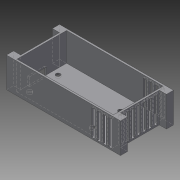
# Autodesk Inventor part: case body
Saved by Autodesk Inventor 2015 (Build 190159000, 159)
## iProperties
Created: 2019-05-19
Part Number: case body
Material: Generic
Document SubType Name: Modeling
Designer: Toby
Density: 1 g/cm^3
Appearance: Default
Author: Toby
Autodesk Inventor part; units mm, degrees
ref_plane "YZ Plane" through (0, 0, 0) normal (1, 0, 0) x (0, 1, 0)
ref_plane "XZ Plane" through (0, 0, 0) normal (0, 1, 0) x (-1, 0, 0)
ref_plane "XY Plane" through (0, 0, 0) normal (0, 0, 1) x (1, 0, 0)
sketch "Sketch1" plane through (0, 0, 0) normal (0, 0, 1) x (1, 0, 0)
  line L0 (-48.8389, 19.9623) -> (19.1611, 19.9623)
  line L1 (19.1611, 19.9623) -> (19.1611, -15.0377)
  line L2 (19.1611, -15.0377) -> (-48.8389, -15.0377)
  line L3 (-48.8389, -15.0377) -> (-48.8389, 19.9623)
  line L4 (-50.0389, 21.1623) -> (20.3611, 21.1623)
  line L5 (20.3611, 21.1623) -> (20.3611, -16.2377)
  line L6 (20.3611, -16.2377) -> (-50.0389, -16.2377)
  line L7 (-50.0389, -16.2377) -> (-50.0389, 21.1623)
  point P0 (0, 0)
  dimension "d0" = 35
  dimension "d1" = 68
  dimension "d2" = 1.2
  dimension "d3" = 1.2
  dimension "d4" = 1.2
  dimension "d5" = 1.2
  constraints: 16 end point, 4 parallel, 2 horizontal, 2 perpendicular
  measures "d0" distance between parallel lines of L2 L0
  measures "d1" distance of L0.start L0.end
  measures "d2" distance between parallel lines of L0 L4
  measures "d3" distance between parallel lines of L6 L2
  measures "d4" distance between parallel lines of L7 L3
  measures "d5" distance between parallel lines of L1 L5
extrude "Extrusion1" add sketch "Sketch1" along normal blind 20
sketch "Sketch2" plane through (0, 0, 0) normal (0, 0, -1) x (-1, 0, 0)
  line L0 (-20.3611, 21.1623) -> (50.0389, 21.1623)
  line L1 (50.0389, 21.1623) -> (50.0389, -16.2377)
  line L2 (50.0389, -16.2377) -> (-20.3611, -16.2377)
  line L3 (-20.3611, -16.2377) -> (-20.3611, 21.1623)
  point P0 (0, 0)
  constraints: 8 end point, 2 parallel, 1 horizontal, 1 perpendicular
extrude "Extrusion2" add sketch "Sketch2" along normal blind 1.2
sketch "Sketch3" plane through (-50.0389, -16.2377, 20) normal (-1, 0, 0) x (0, 0, 1)
  line L0 (-21.2, 0) -> (-21.2, 37.4) projected
  line L1 (-21.2, 22) -> (-15.2, 22)
  line L2 (-15.2, 22) -> (-15.2, 10)
  line L3 (-15.2, 10) -> (-21.2, 10)
  line L4 (-21.2, 10) -> (-21.2, 22)
  line L5 (0, 0) -> (-21.2, 0) projected
  point P0 (-20, 16.2377)
  dimension "d10" = 10
  dimension "d11" = 22
  dimension "d12" = 6
  constraints: 8 end point, 2 parallel, 1 horizontal, 1 perpendicular, 1 point on line
  measures "d10" distance between parallel lines of L5 L3
  measures "d11" distance between parallel lines of L5 L1
  measures "d12" distance between parallel lines of L0 L2
extrude "Extrusion3" cut sketch "Sketch3" against normal blind 1.2
sketch "Sketch4" plane through (0, 0, 0) normal (0, 0, 1) x (1, 0, 0)
  line L0 (19.1611, -15.0377) -> (-48.8389, -15.0377) projected
  line L1 (-48.8389, -15.0377) -> (-48.8389, 19.9623) projected
  circle A0 centre (-44.8389, 9.9623) radius 2.5
  circle A1 centre (-44.8389, -10.0377) radius 2.5
  circle A2 centre (-0.8389, 9.9623) radius 2.5
  circle A3 centre (-0.8389, -10.0377) radius 2.5
  point P0 (0, 0)
  dimension "d15" = 5
  dimension "d16" = 25
  dimension "d17" = 4
  dimension "d18" = 4
  dimension "d19" = 44
  dimension "d20" = 44
  dimension "d21" = 5
  dimension "d22" = 25
  dimension "d23" = 5
  dimension "d24" = 5
  dimension "d25" = 5
  dimension "d26" = 5
  constraints: 4 centre point, 4 coincident
  measures "d15" distance from line of L0 point (-44.839, -10.038)
  measures "d16" distance from line of L0 point (-44.839, 9.962)
  measures "d17" distance from line of L1 point (-44.839, 9.962)
  measures "d18" distance from line of L1 point (-44.839, -10.038)
  measures "d19" distance of point (-44.839, 9.962) point (-0.839, 9.962)
  measures "d20" distance of point (-44.839, -10.038) point (-0.839, -10.038)
  measures "d21" distance from line of L0 point (-0.839, -10.038)
  measures "d22" distance from line of L0 point (-0.839, 9.962)
  measures "d23" diameter of A0
  measures "d24" diameter of A1
  measures "d25" diameter of A2
  measures "d26" diameter of A3
hole "Hole1" at (-44.8389, -10.0377, 0) at (-44.8389, 9.9623, 0) at (-0.8389, 9.9623, 0) at (-0.8389, -10.0377, 0) direction (0, 0, -1) diameter 3 depth 8 tip angle 118
sketch "Sketch5" plane through (0, 0, 20) normal (0, 0, 1) x (1, 0, 0)
  line L0 (-50.0389, 21.1623) -> (-55.0389, 21.1623)
  line L1 (-55.0389, 21.1623) -> (-55.0389, 16.1623)
  line L2 (-55.0389, 16.1623) -> (-50.0389, 16.1623)
  line L3 (-50.0389, 16.1623) -> (-50.0389, 21.1623)
  line L4 (-50.0389, -16.2377) -> (-55.0389, -16.2377)
  line L5 (-55.0389, -16.2377) -> (-55.0389, -11.2377)
  line L6 (-55.0389, -11.2377) -> (-50.0389, -11.2377)
  line L7 (-50.0389, -11.2377) -> (-50.0389, -16.2377)
  line L8 (20.3611, -16.2377) -> (25.3611, -16.2377)
  line L9 (25.3611, -16.2377) -> (25.3611, -11.2377)
  line L10 (25.3611, -11.2377) -> (20.3611, -11.2377)
  line L11 (20.3611, -11.2377) -> (20.3611, -16.2377)
  line L12 (20.3611, 21.1623) -> (25.3611, 21.1623)
  line L13 (25.3611, 21.1623) -> (25.3611, 16.1623)
  line L14 (25.3611, 16.1623) -> (20.3611, 16.1623)
  line L15 (20.3611, 16.1623) -> (20.3611, 21.1623)
  line L16 (20.3611, -16.2377) -> (20.3611, 21.1623) projected
  point P0 (0, 0)
  dimension "d34" = 5
  dimension "d35" = 5
  dimension "d36" = 5
  dimension "d37" = 5
  dimension "d38" = 5
  dimension "d39" = 5
  dimension "d40" = 5
  dimension "d41" = 5
  constraints: 32 end point, 8 parallel, 4 horizontal, 4 perpendicular, 3 point on line, 1 collinear
  measures "d34" distance of L2.end L1.end
  measures "d35" distance of L1.end L0.end
  measures "d36" distance of L5.end L6.end
  measures "d37" distance of L4.end L5.end
  measures "d38" distance of L10.end L9.end
  measures "d39" distance of L9.end L8.end
  measures "d40" distance of L13.end L14.end
  measures "d41" distance of L12.end L13.end
extrude "Extrusion4" add sketch "Sketch5" against normal blind 21.2
sketch "Sketch6" plane through (20.3611, -11.2377, -1.2) normal (1, 0, 0) x (0, 0, -1)
  line L0 (-21.2, 0) -> (0, 0) projected
  line L1 (-19.2, 0) -> (-1.2, 0)
  line L2 (-1.2, 0) -> (-1.2, 2)
  line L3 (-1.2, 2) -> (-19.2, 2)
  line L4 (-19.2, 2) -> (-19.2, 0)
  line L5 (-1.2, -3.8) -> (-1.2, 31.2) projected
  line L6 (-19.2, 4) -> (-1.2, 4)
  line L7 (-1.2, 4) -> (-1.2, 6)
  line L8 (-1.2, 6) -> (-19.2, 6)
  line L9 (-19.2, 6) -> (-19.2, 4)
  line L10 (-19.2, 8) -> (-1.2, 8)
  line L11 (-1.2, 8) -> (-1.2, 10)
  line L12 (-1.2, 10) -> (-19.2, 10)
  line L13 (-19.2, 10) -> (-19.2, 8)
  line L14 (-19.2, 12) -> (-1.2, 12)
  line L15 (-1.2, 12) -> (-1.2, 14)
  line L16 (-1.2, 14) -> (-19.2, 14)
  line L17 (-19.2, 14) -> (-19.2, 12)
  line L18 (-19.2, 16) -> (-1.2, 16)
  line L19 (-1.2, 16) -> (-1.2, 18)
  line L20 (-1.2, 18) -> (-19.2, 18)
  line L21 (-19.2, 18) -> (-19.2, 16)
  line L22 (-19.2, 20) -> (-1.2, 20)
  line L23 (-1.2, 20) -> (-1.2, 22)
  line L24 (-1.2, 22) -> (-19.2, 22)
  line L25 (-19.2, 22) -> (-19.2, 20)
  line L26 (-19.2, 24) -> (-1.2, 24)
  line L27 (-1.2, 24) -> (-1.2, 26)
  line L28 (-1.2, 26) -> (-19.2, 26)
  line L29 (-19.2, 26) -> (-19.2, 24)
  point P0 (-1.2, 11.2377)
  point P1 (-19.2, -2)
  dimension "d44" = 18
  dimension "d45" = 2
  dimension "d46" = 2
  dimension "d47" = 18
  dimension "d48" = 2
  dimension "d49" = 18
  dimension "d50" = 2
  dimension "d51" = 18
  dimension "d52" = 2
  dimension "d53" = 18
  dimension "d54" = 2
  dimension "d55" = 18
  dimension "d56" = 2
  dimension "d57" = 18
  dimension "d58" = 2
  constraints: 56 end point, 14 parallel, 7 horizontal, 7 perpendicular, 1 collinear, 1 point on line
  measures "d44" distance of L3.end L2.end
  measures "d45" distance of L2.end L1.end
  measures "d46" distance from line of L0 point (-19.2, -2)
  measures "d47" distance of L9.start L8.start
  measures "d48" distance of L8.start L6.end
  measures "d49" distance of L13.start L12.start
  measures "d50" distance of L12.start L10.end
  measures "d51" distance of L17.start L16.start
  measures "d52" distance of L16.start L14.end
  measures "d53" distance of L21.start L20.start
  measures "d54" distance of L20.start L18.end
  measures "d55" distance of L25.start L24.start
  measures "d56" distance of L24.start L22.end
  measures "d57" distance of L29.start L28.start
  measures "d58" distance of L28.start L26.end
extrude "Extrusion5" cut sketch "Sketch6" against normal blind 1.2
sketch "Sketch7" plane through (-55.0389, 21.1623, 20) normal (0, 1, 0) x (1, 0, 0)
  line L0 (74.2, 20) -> (72.2, 20)
  line L1 (72.2, 20) -> (72.2, 2)
  line L2 (72.2, 2) -> (74.2, 2)
  line L3 (74.2, 2) -> (74.2, 20)
  line L4 (70.2, 20) -> (68.2, 20)
  line L5 (68.2, 20) -> (68.2, 2)
  line L6 (68.2, 2) -> (70.2, 2)
  line L7 (70.2, 2) -> (70.2, 20)
  line L8 (66.2, 20) -> (64.2, 20)
  line L9 (64.2, 20) -> (64.2, 2)
  line L10 (64.2, 2) -> (66.2, 2)
  line L11 (66.2, 2) -> (66.2, 20)
  line L12 (62.2, 20) -> (60.2, 20)
  line L13 (60.2, 20) -> (60.2, 2)
  line L14 (60.2, 2) -> (62.2, 2)
  line L15 (62.2, 2) -> (62.2, 20)
  point P0 (55.0389, 20)
  point P1 (76.2, 2)
  dimension "d61" = 2
  dimension "d62" = 18
  dimension "d63" = 2
  dimension "d64" = 2
  dimension "d65" = 18
  dimension "d66" = 2
  dimension "d67" = 18
  dimension "d68" = 2
  dimension "d69" = 18
  constraints: 32 end point, 8 parallel, 4 horizontal, 4 perpendicular
  measures "d61" distance of L2.end L1.end
  measures "d62" distance of L1.end L0.end
  measures "d63" distance from line of L3 point (76.2, 2)
  measures "d64" distance of L7.start L5.end
  measures "d65" distance of L5.end L5.start
  measures "d66" distance of L11.start L9.end
  measures "d67" distance of L9.end L9.start
  measures "d68" distance of L15.start L13.end
  measures "d69" distance of L13.end L13.start
extrude "Extrusion6" cut sketch "Sketch7" against normal blind 100
body "Solid1"
